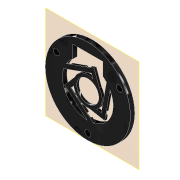
# Autodesk Inventor part: 50_ETL_Spring_v0
Saved by Autodesk Inventor 2022 (Build 260153000, 153)
## iProperties
Created: 2021-12-31
Part Number: 50_ETL_Spring_v0
Material: Generisch
Document SubType Name: Modeling
Designer: diederichbenedict
Density: 1 g/cm^3
Appearance: Schwarz
Mass: 1.84042 g
Surface Area: 24.047 cm^2
Volume: 1.84042 cm^3
Author: diederichbenedict
Autodesk Inventor part; units mm, degrees
ref_plane "YZ Plane" through (0, 0, 0) normal (1, 0, 0) x (0, 1, 0)
ref_plane "XZ Plane" through (0, 0, 0) normal (0, 1, 0) x (-1, 0, 0)
ref_plane "XY Plane" through (0, 0, 0) normal (0, 0, 1) x (1, 0, 0)
ref_plane "Arbeitsebene1" through (0, 0, 0) normal (0, 0, 1) x (1, 0, 0)
sketch "Skizze1" plane through (0, 0, 0) normal (0, 0, 1) x (1, 0, 0)
  circle A0 centre (-27.5894, 8.25) radius 1.4 projected
  circle A1 centre (-13.3, -16.5) radius 1.4 projected
  circle A2 centre (0.9894, 8.25) radius 1.4 projected
  line L0 (-20.05, 11.6913) -> (-20.05, 15.1) projected
  line L1 (-20.05, 15.1) -> (-6.55, 15.1) projected
  line L2 (-6.55, 15.1) -> (-6.55, 11.6913) projected
  circle A3 centre (-13.3, 0) radius 19.3 projected
  circle A4 centre (-13.3, 0) radius 11.5
  line L3 (-6.55, 11.4598) -> (-6.55, 9.3106)
  line L4 (-20.05, 11.4598) -> (-20.05, 9.3106)
  arc A5 (-20.05, 11.6913) -> (-6.55, 11.6913) centre (-13.3, 0) ccw projected
  line L5 (-6.55, 11.6913) -> (-6.55, 11.4598)
  line L6 (-20.05, 11.6913) -> (-20.05, 11.4598)
  dimension "d0" = 23
  constraints: 8 end point, 2 parallel, 2 point on circle, 2 vertical, 1 centre point, 1 coincident
  measures "d0" diameter of A4
extrude "Extrusion1" add sketch "Skizze1" along normal blind 2 contours L6 L4 A4 L3 L5 A5 | A3
sketch "Skizze2" plane through (-13.3, 0, 2) normal (0, 0, 1) x (1, 0, 0)
  circle A0 centre (0, 0) radius 19.3 projected
  circle A1 centre (14.2894, 8.25) radius 1.4 projected
  circle A2 centre (0, -16.5) radius 1.4 projected
  circle A3 centre (-14.2894, 8.25) radius 1.4 projected
  circle A4 centre (0, 0) radius 5 projected
  arc A5 (2.8009, 5.3061) -> (-2.8009, 5.3061) centre (0, 0) ccw construction
  line L0 (2.8009, 5.3061) -> (6.25, 5.3061) construction
  line L1 (6.25, 5.3061) -> (6.25, 14.6) construction
  line L2 (6.25, 14.6) -> (-6.25, 14.6) construction
  line L3 (-6.25, 14.6) -> (-6.25, 5.3061) construction
  line L4 (-6.25, 5.3061) -> (-2.8009, 5.3061) construction
  circle A6 centre (0, 0) radius 6.5
  arc A7 (-6.75, 9.3106) -> (6.75, 9.3106) centre (0, 0) ccw projected
  line L5 (8.462, 7.7874) -> (6.0645, -5.4052)
  line L6 (6.0645, -5.4052) -> (8.0323, -5.7628)
  line L7 (8.0323, -5.7628) -> (10.0842, 5.528)
  line L8 (8.0323, -5.7628) -> (7.6747, -7.7305)
  line L9 (7.6747, -7.7305) -> (3.738, -7.0151)
  line L10 (3.738, -7.0151) -> (4.0956, -5.0474)
  line L11 (4.0956, -5.0474) -> (8.0323, -5.7628)
  line L12 (3.738, -7.0151) -> (0.6972, -6.4625)
  line L13 (6.75, 15.1) -> (6.75, 9.3106) projected
  line L14 (6.75, 9.3106) -> (6.75, 11.6913)
  line L15 (-6.75, 9.3106) -> (-6.75, 11.6913)
  arc A8 (-6.75, 11.6913) -> (6.75, 11.6913) centre (0, 0) ccw projected
  point P0 (13.3, 0)
  dimension "d3" = 13
  dimension "d4" = 2
  dimension "d5" = 2
  constraints: 20 end point, 4 point on circle, 3 perpendicular, 2 parallel, 2 vertical, 1 centre point, 1 coincident, 1 collinear, 1 point on line
  measures "d3" diameter of A6
  measures "d4" distance of L5.end L6.end
  measures "d5" distance between parallel lines of L9 L11
extrude "Extrusion2" add sketch "Skizze2" against normal blind 1 contours A6 | A6 L10 L12 | L11 L6 L8 L9 L10 | L5 A7 L7 L6
sketch "Skizze3" plane through (-13.3, 0, 1) normal (0, 0, 1) x (1, 0, 0)
  circle A0 centre (0, 0) radius 19.3 projected
  circle A1 centre (14.2894, 8.25) radius 1.4 projected
  circle A2 centre (0, -16.5) radius 1.4 projected
  circle A3 centre (-14.2894, 8.25) radius 1.4 projected
  line L0 (6.0645, -5.4052) -> (8.462, 7.7874) projected
  line L1 (7.6747, -7.7305) -> (10.0842, 5.528) projected
  line L2 (6.0645, -5.4052) -> (8.0323, -5.7628)
  line L3 (8.0323, -5.7628) -> (8.3899, -3.795)
  line L4 (8.3899, -3.795) -> (6.4221, -3.4374)
  line L5 (6.4221, -3.4374) -> (6.0645, -5.4052)
  line L6 (10.0842, 5.528) -> (8.1164, 5.8856)
  line L7 (8.1164, 5.8856) -> (7.7588, 3.9179)
  line L8 (7.7588, 3.9179) -> (9.7266, 3.5603)
  line L9 (9.7266, 3.5603) -> (10.0842, 5.528)
  point P0 (13.3, 0)
  dimension "d8" = 2
  dimension "d9" = 2
  constraints: 16 end point, 4 parallel, 3 perpendicular, 1 point on line
  measures "d8" distance of L3.end L2.end
  measures "d9" distance of L7.end L6.end
extrude "Extrusion3" cut sketch "Skizze3" along normal blind 0.7 contours L0 L4 L1 L2 | L0 L6 L1 L8
pattern_circular "Runde Anordnung1" count 3 over 360 about axis through (-13.3, 0, 2) along (0, 0, -1) of "Extrusion3", "Extrusion2"
